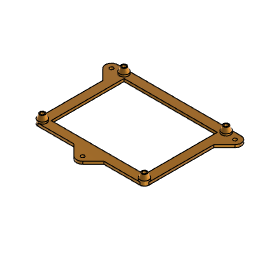
Duet WiFi Standoff (Autodesk Fusion 360 design; units mm, degrees)
Autodesk Fusion 360 part; units mm, degrees
sketch "Sketch1" plane through (0, 0, 0) normal (0, 0, 1) x (1, 0, 0)
  line L0 (0, 0) -> (123, 0) construction
  line L1 (123, 0) -> (123, -100) construction
  line L2 (123, -100) -> (0, -100) construction
  line L3 (0, -100) -> (0, 0) construction
  line L4 (4, -4) -> (119, -4) construction
  line L5 (119, -4) -> (119, -96) construction
  line L6 (119, -96) -> (4, -96) construction
  line L7 (4, -96) -> (4, -4) construction
  line L8 (0, -50) -> (4, -50) construction
  line L9 (61.5, 0) -> (61.5, -4) construction
  line L10 (0, -100) -> (123, 0) construction
  line L11 (0, 0) -> (123, -100) construction
  circle A0 centre (119, -4) radius 5
  circle A1 centre (4, -4) radius 5
  circle A2 centre (4, -96) radius 5
  circle A3 centre (119, -96) radius 5
  line L12 (-8, 1) -> (131, 1)
  line L13 (124, -4) -> (124, -96)
  line L14 (4, -101) -> (119, -101)
  line L15 (-1, -4) -> (-1, -96)
  line L16 (4, -9) -> (119, -9)
  line L17 (114, -4) -> (114, -96)
  line L18 (119, -91) -> (4, -91)
  line L19 (9, -4) -> (9, -96)
  circle A4 centre (131, -6) radius 2
  circle A5 centre (-8, -6) radius 2
  circle A6 centre (61.5, -108) radius 2
  line L20 (61.5, -101) -> (61.5, -115) construction
  circle A7 centre (131, -6) radius 7
  line L21 (135.9497, -10.9497) -> (124, -22.8995)
  circle A8 centre (-8, -6) radius 7
  line L22 (-12.9497, -10.9497) -> (-1, -22.8995)
  circle A9 centre (61.5, -108) radius 7
  line L23 (66.4497, -112.9497) -> (78.3995, -101)
  line L24 (44.6005, -101) -> (56.5503, -112.9497)
  point P0 (61.5, -96)
  point P1 (119, -50)
  dimension "d1" = 123
  dimension "d2" = 100
  dimension "d3" = 92
  dimension "d7" = 4
  dimension "d8" = 4
  dimension "d9" = 4
  dimension "d10" = 4
  dimension "d60" = 10
  dimension "d62" = 4
  dimension "d63" = 4
  dimension "d64" = 4
  dimension "d83" = 45
  dimension "d85" = 45
  dimension "d87" = 45
  dimension "d89" = 5
  dimension "d90" = 10
  dimension "d91" = 115
  dimension "d96" = 0
  dimension "d97" = 0
  dimension "d98" = 0
  dimension "d99" = 0
  constraint horizontal L0
  constraint vertical L1
  constraint horizontal L2
  constraint vertical L3
  constraint coincident L0.start L3.end
  constraint horizontal L4
  constraint vertical L5
  constraint horizontal L6
  constraint vertical L7
  constraint midpoint L3 L8.start
  constraint perpendicular L7 L8
  constraint midpoint L7 L8.end
  constraint midpoint L0 L9.start
  constraint perpendicular L4 L9
  constraint midpoint L4 L9.end
  constraint midpoint L6 P0
  constraint midpoint L5 P1
  constraint coincident L4.end L5.start
  constraint coincident L4.start L7.end
  constraint coincident L6.end L7.start
  constraint coincident L5.end L6.start
  constraint equal A0 A3
  constraint equal A0 A1
  constraint equal A1 A2
  constraint tangent A1 L12
  constraint tangent A0 L12
  constraint coincident A0 L13.start
  constraint tangent A0 L13
  constraint coincident A3 L13.end
  constraint tangent A3 L13
  constraint coincident A2 L14.start
  constraint tangent A2 L14
  constraint coincident A3 L14.end
  constraint tangent A3 L14
  constraint coincident A1 L15.start
  constraint tangent A1 L15
  constraint coincident A2 L15.end
  constraint tangent A2 L15
  constraint coincident A1 L16.start
  constraint tangent A1 L16
  constraint coincident A0 L16.end
  constraint coincident L5 L16.end
  constraint coincident A0 L17.start
  constraint tangent A0 L17
  constraint coincident L6 L17.end
  constraint coincident A3 L17.end
  constraint coincident A3 L18.start
  constraint tangent A3 L18
  constraint coincident L7 L18.end
  constraint coincident A2 L18.end
  constraint coincident A1 L19.start
  constraint tangent A1 L19
  constraint coincident L6 L19.end
  constraint coincident A2 L19.end
  constraint midpoint A6.centre L20
  constraint concentric A4 A7
  constraint tangent L13 A7
  constraint tangent L12 A7
  constraint coincident L12.end A7
  constraint coincident A7 L21.start
  constraint tangent A7 L21
  constraint coincident L13 L21.end
  constraint concentric A5 A8
  constraint tangent L15 A8
  constraint tangent L12 A8
  constraint coincident L12.start A8
  constraint coincident A8 L22.start
  constraint tangent A8 L22
  constraint coincident L15 L22.end
  constraint concentric A6 A9
  constraint tangent L14 A9
  constraint midpoint L14 L20.start
  constraint perpendicular L14 L20
  constraint coincident A9 L23.start
  constraint tangent A9 L23
  constraint coincident L14 L23.end
  constraint coincident L14 L24.start
  constraint coincident A9 L24.end
  constraint tangent A9 L24
  constraint symmetric L20 L23.end L24.start
  constraint equal A7 A8
  constraint equal A7 A9
  measures "d1" distance of L0.start L0.end
  measures "d2" distance of L0.start L2.end
  measures "d3" distance of L4.start L6.end
  measures "d7" horizontal distance of L0.end L4.end
  measures "d8" vertical distance of L0.end L4.end
  measures "d9" vertical distance of L1.end L5.end
  measures "d10" horizontal distance of L2.end L6.end
  measures "d60" diameter of A0
  measures "d62" diameter of A4
  measures "d63" diameter of A5
  measures "d64" diameter of A6
  measures "d83" angle of L13 L21
  measures "d85" angle of L15 L22
  measures "d87" angle of L14 L23
  measures "d89" distance of A4 A7
  measures "d91" distance of L4.start L4.end
extrude "Extrude1" add sketch "Sketch1" along normal blind 3 contours A0 | A0 A1 L12 L16 L17 L19 | A0 L16 L17 | A0 A3 L13 L16 L17 L18 | A0 L12 L13 A7 | A1 | A1 L12 L15 A8 | A7 | A1 A2 L15 L16 L18 L19 | A1 L16 L19 | A3 L17 L18 | A2 A3 L14 L17 L18 L19 | L13 A7 L21 | A8 | A2 L18 L19 | A3 | L15 A8 L22 | A2 | L14 A9 L23 | L14 A9 L24 | A9
sketch "Sketch2" plane through (0, 0, 3) normal (0, 0, 1) x (-1, 0, 0)
  circle A0 centre (-119, 96) radius 5
  circle A1 centre (-119, 4) radius 5
  circle A2 centre (-4, 4) radius 5
  circle A3 centre (-4, 96) radius 5
extrude "Extrude5" add sketch "Sketch2" along normal blind 2
ref_plane "WorkPlane1" through (4, -4, 10) normal (0, 0, 1) x (-1, 0, 0)
sketch "Sketch4" plane through (4, -4, 10) normal (0, 0, 1) x (1, 0, 0)
  circle A0 centre (115, 0) radius 5 construction
  circle A1 centre (0, 0) radius 5 construction
  circle A2 centre (115, -92) radius 5 construction
  circle A3 centre (0, -92) radius 5 construction
  circle A4 centre (0, 0) radius 3
  circle A5 centre (115, 0) radius 3
  circle A6 centre (115, -92) radius 3
  circle A7 centre (0, -92) radius 3
  dimension "d72" = 6
  constraint concentric A1 A4
  constraint concentric A0 A5
  constraint concentric A2 A6
  constraint concentric A3 A7
  constraint equal A4 A6
  constraint equal A5 A6
  constraint equal A4 A7
  measures "d72" diameter of A4
loft "Loft1" add profiles "Sketch4" section 1 face at (5.1043, -98.6306, 5) section 2 contours A7
pattern_linear "R-Pattern1" count 2 spacing 115 along (1, 0, 0) count 2 spacing 92 along (0, 1, 0) of "Loft1"
hole "Hole3" at (4, -96, 0) at (119, -96, 0) at (119, -4, 0) at (4, -4, 0) direction (0, 0, 1) diameter 4 depth 23 tip angle 118 counterbore diameter 6.5 counterbore depth 4
chamfer "Chamfer1" distance 1 angle 45 4 edges at (7.0301, -94.8247, 4) (122.0301, -94.8247, 4) (122.0301, -2.8247, 4) (7.0301, -2.8247, 4)
equation "d29 = 14 mm"
equation "d31 = d29"
equation "d85 = d83"
named bodies: "Duet Wifi Standoff"
